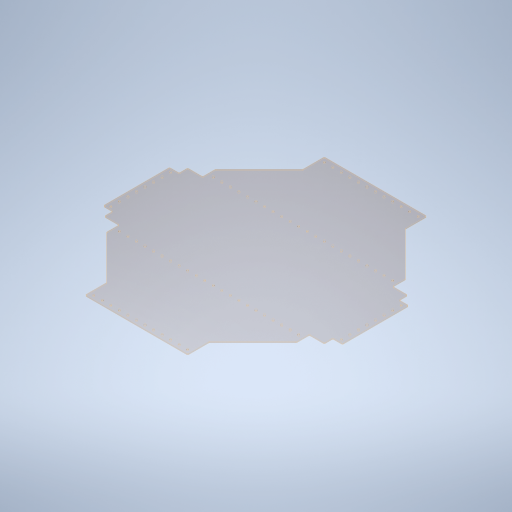
# Autodesk Inventor part: DB1-005
Saved by Autodesk Inventor 2023.4 (Build 274418000, 418)
## iProperties
Created: 2025-01-13
Part Number: DB1-005
Material: Polycarbonate, Smoke
Document SubType Name: Modeling
Designer: mavericks
Density: 1.2 g/cm^3
Appearance: Polycarbonate - Smoked
Author: mavericks
Autodesk Inventor part; units mm, degrees
ref_plane "YZ Plane" through (0, 0, 0) normal (1, 0, 0) x (0, 1, 0)
ref_plane "XZ Plane" through (0, 0, 0) normal (0, 1, 0) x (-1, 0, 0)
ref_plane "XY Plane" through (0, 0, 0) normal (0, 0, 1) x (1, 0, 0)
sketch "Sketch1" plane through (0, 0, 0) normal (0, 1, 0) x (-1, 0, 0)
  line L0 (355.6, 355.6) -> (-355.6, 355.6)
  line L1 (-355.6, 355.6) -> (-355.6, -355.6)
  line L2 (-355.6, -355.6) -> (355.6, -355.6)
  line L3 (355.6, -355.6) -> (355.6, 355.6)
  line L4 (355.6, 355.6) -> (-355.6, -355.6) construction
  line L5 (-355.6, 355.6) -> (355.6, -355.6) construction
  line L6 (152.4, 355.6) -> (152.4, 292.1)
  line L7 (152.4, 292.1) -> (292.1, 152.4)
  line L8 (292.1, 152.4) -> (355.6, 152.4)
  line L9 (-152.4, 292.1) -> (-152.4, 355.6)
  line L10 (-292.1, 152.4) -> (-152.4, 292.1)
  line L11 (-355.6, 152.4) -> (-292.1, 152.4)
  line L12 (-292.1, -152.4) -> (-355.6, -152.4)
  line L13 (-152.4, -292.1) -> (-292.1, -152.4)
  line L14 (-152.4, -355.6) -> (-152.4, -292.1)
  line L15 (152.4, -292.1) -> (152.4, -355.6)
  line L16 (292.1, -152.4) -> (152.4, -292.1)
  line L17 (355.6, -152.4) -> (292.1, -152.4)
  point P0 (0, 0)
  dimension "d0" = 711.2
  dimension "d1" = 711.2
  dimension "d2" = 63.5
  dimension "d3" = 203.2
  dimension "d6" = 360
  constraints: 36 end point, 4 perpendicular, 2 midpoint, 2 parallel, 2 point on line, 1 horizontal, 1 vertical, 29 other
  measures "d0" distance of L2.end L1.end
  measures "d1" distance of L1.end L0.end
  measures "d2" distance of L6.end L6.start
  measures "d3" distance of L0.start L6.start
extrude "Extrusion1" add sketch "Sketch1" along normal blind 3.175 contours L6 L7 L8 L3 L17 L16 L15 L2 L14 L13 L12 L1 L11 L10 L9 L0
sketch "Sketch2" plane through (0, 3.175, 0) normal (0, 1, 0) x (1, 0, 0)
  line L0 (-355.6, 152.4) -> (-355.6, -152.4) construction
  line L1 (152.4, 355.6) -> (-152.4, 355.6) construction
  line L2 (-152.4, -355.6) -> (152.4, -355.6) construction
  line L3 (355.6, -152.4) -> (355.6, 152.4) construction
  line L4 (-292.1, 152.4) -> (-355.6, 152.4) construction
  line L5 (-152.4, -292.1) -> (-152.4, -355.6) construction
  point P0 (0, 0)
  point P1 (-139.7, -342.9)
  point P2 (-139.7, 342.9)
  point P3 (342.9, 139.7)
  point P4 (-342.9, 139.7)
  point P5 (-114.3, -342.9)
  point P6 (-114.3, 342.9)
  point P7 (-88.9, -342.9)
  point P8 (-88.9, 342.9)
  point P9 (-63.5, -342.9)
  point P10 (-63.5, 342.9)
  point P11 (-38.1, -342.9)
  point P12 (-38.1, 342.9)
  point P13 (-12.7, -342.9)
  point P14 (-12.7, 342.9)
  point P15 (12.7, -342.9)
  point P16 (12.7, 342.9)
  point P17 (38.1, -342.9)
  point P18 (38.1, 342.9)
  point P19 (63.5, -342.9)
  point P20 (63.5, 342.9)
  point P21 (88.9, -342.9)
  point P22 (88.9, 342.9)
  point P23 (114.3, -342.9)
  point P24 (114.3, 342.9)
  point P25 (139.7, -342.9)
  point P26 (139.7, 342.9)
  point P27 (-342.9, 114.3)
  point P28 (342.9, 114.3)
  point P29 (-342.9, 88.9)
  point P30 (342.9, 88.9)
  point P31 (-342.9, 63.5)
  point P32 (342.9, 63.5)
  point P33 (-342.9, 38.1)
  point P34 (342.9, 38.1)
  point P35 (-342.9, 12.7)
  point P36 (342.9, 12.7)
  point P37 (-342.9, -12.7)
  point P38 (342.9, -12.7)
  point P39 (-342.9, -38.1)
  point P40 (342.9, -38.1)
  point P41 (-342.9, -63.5)
  point P42 (342.9, -63.5)
  point P43 (-342.9, -88.9)
  point P44 (342.9, -88.9)
  point P45 (-342.9, -114.3)
  point P46 (342.9, -114.3)
  point P47 (-342.9, -139.7)
  point P48 (342.9, -139.7)
  dimension "d10" = 12.7
  dimension "d11" = 12.7
  dimension "d12" = 12.7
  dimension "d13" = 12.7
  dimension "d14" = 12.7
  dimension "d15" = 12.7
  dimension "d18" = 25.4
  dimension "d25" = 25.4
  constraints: 1 horizontal, 1 horizontal alignment, 1 vertical, 1 vertical alignment, 44 other
  measures "d10" distance from line of L0 point (-342.9, 139.7)
  measures "d11" distance from line of L1 point (-139.7, 342.9)
  measures "d12" distance from line of L2 point (-139.7, -342.9)
  measures "d13" distance from line of L3 point (342.9, 139.7)
  measures "d14" distance from line of L4 point (-342.9, 139.7)
  measures "d15" distance from line of L5 point (-139.7, -342.9)
  measures "d18" distance of point (-139.7, -342.9) point (-114.3, -342.9)
  measures "d25" distance of point (-342.9, 139.7) point (-342.9, 114.3)
hole "Hole1" at (-139.7, 3.175, 342.9) at (-139.7, 3.175, -342.9) at (342.9, 3.175, -139.7) at (-342.9, 3.175, -139.7) at (-114.3, 3.175, 342.9) at (-114.3, 3.175, -342.9) at (-88.9, 3.175, 342.9) at (-88.9, 3.175, -342.9) at (-63.5, 3.175, 342.9) at (-63.5, 3.175, -342.9) at (-38.1, 3.175, 342.9) at (-38.1, 3.175, -342.9) at (-12.7, 3.175, 342.9) at (-12.7, 3.175, -342.9) at (12.7, 3.175, 342.9) at (12.7, 3.175, -342.9) at (38.1, 3.175, 342.9) at (38.1, 3.175, -342.9) at (63.5, 3.175, 342.9) at (63.5, 3.175, -342.9) at (88.9, 3.175, 342.9) at (88.9, 3.175, -342.9) at (114.3, 3.175, 342.9) at (114.3, 3.175, -342.9) at (139.7, 3.175, 342.9) at (139.7, 3.175, -342.9) at (-342.9, 3.175, -114.3) at (342.9, 3.175, -114.3) at (-342.9, 3.175, -88.9) at (342.9, 3.175, -88.9) at (-342.9, 3.175, -63.5) at (342.9, 3.175, -63.5) at (-342.9, 3.175, -38.1) at (342.9, 3.175, -38.1) at (-342.9, 3.175, -12.7) at (342.9, 3.175, -12.7) at (-342.9, 3.175, 12.7) at (342.9, 3.175, 12.7) at (-342.9, 3.175, 38.1) at (342.9, 3.175, 38.1) at (-342.9, 3.175, 63.5) at (342.9, 3.175, 63.5) at (-342.9, 3.175, 88.9) at (342.9, 3.175, 88.9) at (-342.9, 3.175, 114.3) at (342.9, 3.175, 114.3) at (-342.9, 3.175, 139.7) at (342.9, 3.175, 139.7) direction (0, -1, 0) diameter 5.1054 end through all clearance for "Flat Head Machine Screw (82)" size "#10" standard "Ansi Unified Screw Threads"
sketch "Sketch3" plane through (0, 3.175, 0) normal (0, 1, 0) x (1, 0, 0)
  circle A0 centre (-342.9, -139.7) radius 2.5527 construction
  circle A1 centre (-342.9, -114.3) radius 2.5527 construction
  circle A2 centre (-342.9, -88.9) radius 2.5527 construction
  circle A3 centre (-342.9, -63.5) radius 2.5527 construction
  circle A4 centre (-342.9, -38.1) radius 2.5527 construction
  circle A5 centre (-342.9, -12.7) radius 2.5527 construction
  circle A6 centre (-342.9, 12.7) radius 2.5527 construction
  circle A7 centre (-342.9, 38.1) radius 2.5527 construction
  circle A8 centre (-342.9, 63.5) radius 2.5527 construction
  circle A9 centre (-342.9, 88.9) radius 2.5527 construction
  circle A10 centre (-342.9, 114.3) radius 2.5527 construction
  circle A11 centre (139.7, -342.9) radius 2.5527 construction
  circle A12 centre (114.3, -342.9) radius 2.5527 construction
  circle A13 centre (88.9, -342.9) radius 2.5527 construction
  circle A14 centre (63.5, -342.9) radius 2.5527 construction
  circle A15 centre (38.1, -342.9) radius 2.5527 construction
  circle A16 centre (12.7, -342.9) radius 2.5527 construction
  circle A17 centre (-12.7, -342.9) radius 2.5527 construction
  circle A18 centre (-38.1, -342.9) radius 2.5527 construction
  circle A19 centre (-63.5, -342.9) radius 2.5527 construction
  circle A20 centre (-88.9, -342.9) radius 2.5527 construction
  circle A21 centre (-114.3, -342.9) radius 2.5527 construction
  circle A22 centre (342.9, 139.7) radius 2.5527 construction
  circle A23 centre (-139.7, -342.9) radius 2.5527 construction
  circle A24 centre (-139.7, 342.9) radius 2.5527 construction
  circle A25 centre (-342.9, 139.7) radius 2.5527 construction
  circle A26 centre (-114.3, 342.9) radius 2.5527 construction
  circle A27 centre (-88.9, 342.9) radius 2.5527 construction
  circle A28 centre (-63.5, 342.9) radius 2.5527 construction
  circle A29 centre (-38.1, 342.9) radius 2.5527 construction
  circle A30 centre (-12.7, 342.9) radius 2.5527 construction
  circle A31 centre (12.7, 342.9) radius 2.5527 construction
  circle A32 centre (38.1, 342.9) radius 2.5527 construction
  circle A33 centre (63.5, 342.9) radius 2.5527 construction
  circle A34 centre (88.9, 342.9) radius 2.5527 construction
  circle A35 centre (114.3, 342.9) radius 2.5527 construction
  circle A36 centre (139.7, 342.9) radius 2.5527 construction
  circle A37 centre (342.9, 114.3) radius 2.5527 construction
  circle A38 centre (342.9, 88.9) radius 2.5527 construction
  circle A39 centre (342.9, 63.5) radius 2.5527 construction
  circle A40 centre (342.9, 38.1) radius 2.5527 construction
  circle A41 centre (342.9, 12.7) radius 2.5527 construction
  circle A42 centre (342.9, -12.7) radius 2.5527 construction
  circle A43 centre (342.9, -38.1) radius 2.5527 construction
  circle A44 centre (342.9, -63.5) radius 2.5527 construction
  circle A45 centre (342.9, -88.9) radius 2.5527 construction
  circle A46 centre (342.9, -114.3) radius 2.5527 construction
  circle A47 centre (342.9, -139.7) radius 2.5527 construction
  line L0 (-152.4, -292.1) -> (-152.4, -355.6) construction
  line L1 (-152.4, -355.6) -> (152.4, -355.6) construction
  line L2 (152.4, -355.6) -> (152.4, -292.1) construction
  line L3 (152.4, -292.1) -> (292.1, -152.4) construction
  line L4 (292.1, -152.4) -> (355.6, -152.4) construction
  line L5 (355.6, -152.4) -> (355.6, 152.4) construction
  line L6 (355.6, 152.4) -> (292.1, 152.4) construction
  line L7 (292.1, 152.4) -> (152.4, 292.1) construction
  line L8 (152.4, 292.1) -> (152.4, 355.6) construction
  line L9 (152.4, 355.6) -> (-152.4, 355.6) construction
  line L10 (-152.4, 355.6) -> (-152.4, 292.1) construction
  line L11 (-152.4, 292.1) -> (-292.1, 152.4) construction
  line L12 (-292.1, 152.4) -> (-355.6, 152.4) construction
  line L13 (-355.6, 152.4) -> (-355.6, -152.4) construction
  line L14 (-355.6, -152.4) -> (-292.1, -152.4) construction
  line L15 (-292.1, -152.4) -> (-152.4, -292.1) construction
  line L16 (-355.6, 152.4) -> (-355.6, -152.4) construction
  line L17 (-355.6, -152.4) -> (-355.6, -98.425)
  line L18 (-355.6, -98.425) -> (-327.025, -98.425)
  line L19 (-327.025, -98.425) -> (-327.025, -123.825)
  line L20 (-327.025, -123.825) -> (-282.575, -123.825)
  line L21 (-355.6, -152.4) -> (-292.1, -152.4) construction
  line L22 (-355.6, -152.4) -> (-282.575, -152.4)
  line L23 (-282.575, -152.4) -> (-282.575, -123.825)
  line L24 (0, 0) -> (-355.6, 0) construction
  line L25 (0, 0) -> (0, 355.6) construction
  line L26 (152.4, 355.6) -> (-152.4, 355.6) construction
  circle A48 centre (-342.9, 139.7) radius 2.5527 construction
  circle A49 centre (-342.9, 114.3) radius 2.5527 construction
  circle A50 centre (-342.9, 88.9) radius 2.5527 construction
  line L27 (-355.6, 152.4) -> (-292.1, 152.4) construction
  line L28 (-355.6, 152.4) -> (-355.6, 98.425)
  line L29 (-355.6, 98.425) -> (-327.025, 98.425)
  line L30 (-327.025, 98.425) -> (-327.025, 123.825)
  line L31 (-327.025, 123.825) -> (-282.575, 123.825)
  line L32 (-355.6, 152.4) -> (-292.1, 152.4) construction
  line L33 (-355.6, 152.4) -> (-282.575, 152.4)
  line L34 (-282.575, 152.4) -> (-282.575, 123.825)
  circle A51 centre (342.9, -139.7) radius 2.5527 construction
  circle A52 centre (342.9, -114.3) radius 2.5527 construction
  circle A53 centre (342.9, -88.9) radius 2.5527 construction
  circle A54 centre (342.9, -63.5) radius 2.5527 construction
  circle A55 centre (342.9, -38.1) radius 2.5527 construction
  circle A56 centre (342.9, -12.7) radius 2.5527 construction
  circle A57 centre (342.9, 12.7) radius 2.5527 construction
  circle A58 centre (342.9, 38.1) radius 2.5527 construction
  circle A59 centre (342.9, 63.5) radius 2.5527 construction
  circle A60 centre (342.9, 88.9) radius 2.5527 construction
  circle A61 centre (342.9, 114.3) radius 2.5527 construction
  circle A62 centre (342.9, 139.7) radius 2.5527 construction
  line L35 (292.1, 152.4) -> (355.6, 152.4) construction
  line L36 (355.6, 152.4) -> (355.6, -152.4) construction
  line L37 (355.6, -152.4) -> (292.1, -152.4) construction
  line L38 (355.6, 152.4) -> (355.6, -152.4) construction
  line L39 (355.6, -152.4) -> (355.6, -98.425)
  line L40 (355.6, -98.425) -> (327.025, -98.425)
  line L41 (327.025, -98.425) -> (327.025, -123.825)
  line L42 (327.025, -123.825) -> (282.575, -123.825)
  line L43 (355.6, -152.4) -> (292.1, -152.4) construction
  line L44 (355.6, -152.4) -> (282.575, -152.4)
  line L45 (282.575, -152.4) -> (282.575, -123.825)
  circle A63 centre (342.9, 139.7) radius 2.5527 construction
  circle A64 centre (342.9, 114.3) radius 2.5527 construction
  line L46 (355.6, 152.4) -> (355.6, 98.425)
  circle A65 centre (342.9, 88.9) radius 2.5527 construction
  line L47 (355.6, 98.425) -> (327.025, 98.425)
  line L48 (327.025, 98.425) -> (327.025, 123.825)
  line L49 (355.6, 152.4) -> (282.575, 152.4)
  line L50 (327.025, 123.825) -> (282.575, 123.825)
  line L51 (282.575, 152.4) -> (282.575, 123.825)
  line L52 (355.6, 152.4) -> (292.1, 152.4) construction
  line L53 (355.6, 152.4) -> (292.1, 152.4) construction
  line L54 (-282.575, -152.4) -> (-282.575, -161.925)
  line L55 (-292.1, -152.4) -> (-152.4, -292.1) construction
  line L56 (-282.575, -161.925) -> (-292.1, -152.4)
  line L57 (-282.575, 152.4) -> (-282.575, 161.925)
  line L58 (-282.575, 161.925) -> (-292.1, 152.4)
  line L59 (282.575, -152.4) -> (282.575, -161.925)
  line L60 (282.575, -161.925) -> (292.1, -152.4)
  line L61 (282.575, 152.4) -> (282.575, 161.925)
  line L62 (282.575, 161.925) -> (292.1, 152.4)
  point P0 (355.6, 0)
  dimension "d39" = 53.975
  dimension "d40" = 28.575
  dimension "d42" = 28.575
  dimension "d43" = 73.025
  constraints: 86 end point, 37 symmetric about line, 18 centre point, 3 point on line, 2 collinear, 2 horizontal, 2 midpoint, 2 perpendicular, 1 vertical, 18 other
  measures "d39" distance of L13.end L17.end
  measures "d40" distance of L17.end L18.end
  measures "d42" distance between parallel lines of L14 L20
  measures "d43" distance from line of L17 L20.end
extrude "Extrusion2" cut sketch "Sketch3" against normal through all
fillet "Fillet1" radius 3.302 28 edges at (-152.4, 1.5875, 355.6) (-152.4, 1.5875, 292.1) (-282.575, 1.5875, 161.925) (-282.575, 1.5875, 123.825) (-327.025, 1.5875, 98.425) (-327.025, 1.5875, 123.825) (-355.6, 1.5875, 98.425) (-355.6, 1.5875, -98.425) (-327.025, 1.5875, -98.425) (-327.025, 1.5875, -123.825) (-282.575, 1.5875, -123.825) (-282.575, 1.5875, -161.925) (-152.4, 1.5875, -292.1) (-152.4, 1.5875, -355.6) (152.4, 1.5875, -292.1) (152.4, 1.5875, -355.6) (282.575, 1.5875, -161.925) (282.575, 1.5875, -123.825) (327.025, 1.5875, -123.825) (327.025, 1.5875, -98.425) (355.6, 1.5875, -98.425) (355.6, 1.5875, 98.425) (327.025, 1.5875, 98.425) (327.025, 1.5875, 123.825) (282.575, 1.5875, 123.825) (282.575, 1.5875, 161.925) (152.4, 1.5875, 292.1) (152.4, 1.5875, 355.6)
sketch "Sketch4" plane through (0, 3.175, 0) normal (0, 1, 0) x (1, 0, 0)
  line L0 (149.098, 355.6) -> (-149.098, 355.6) construction
  line L1 (-149.098, -355.6) -> (149.098, -355.6) construction
  line L2 (355.6, -95.123) -> (355.6, 95.123) construction
  point P0 (0, 0)
  point P1 (266.7, 139.7)
  point P2 (266.7, -139.7)
  point P3 (241.3, 139.7)
  point P4 (241.3, -139.7)
  point P5 (215.9, 139.7)
  point P6 (215.9, -139.7)
  point P7 (190.5, 139.7)
  point P8 (190.5, -139.7)
  point P9 (165.1, 139.7)
  point P10 (165.1, -139.7)
  point P11 (139.7, 139.7)
  point P12 (139.7, -139.7)
  point P13 (114.3, 139.7)
  point P14 (114.3, -139.7)
  point P15 (88.9, 139.7)
  point P16 (88.9, -139.7)
  point P17 (63.5, 139.7)
  point P18 (63.5, -139.7)
  point P19 (38.1, 139.7)
  point P20 (38.1, -139.7)
  point P21 (12.7, 139.7)
  point P22 (12.7, -139.7)
  point P23 (-12.7, 139.7)
  point P24 (-12.7, -139.7)
  point P25 (-38.1, 139.7)
  point P26 (-38.1, -139.7)
  point P27 (-63.5, 139.7)
  point P28 (-63.5, -139.7)
  point P29 (-88.9, 139.7)
  point P30 (-88.9, -139.7)
  point P31 (-114.3, 139.7)
  point P32 (-114.3, -139.7)
  point P33 (-139.7, 139.7)
  point P34 (-139.7, -139.7)
  point P35 (-165.1, 139.7)
  point P36 (-165.1, -139.7)
  point P37 (-190.5, 139.7)
  point P38 (-190.5, -139.7)
  point P39 (-215.9, 139.7)
  point P40 (-215.9, -139.7)
  point P41 (-241.3, 139.7)
  point P42 (-241.3, -139.7)
  point P43 (-266.7, 139.7)
  point P44 (-266.7, -139.7)
  dimension "d45" = 215.9
  dimension "d46" = 215.9
  dimension "d47" = 88.9
  dimension "d50" = 25.4
  constraints: 1 horizontal, 1 vertical alignment, 42 other
  measures "d45" distance from line of L0 point (266.7, 139.7)
  measures "d46" distance from line of L1 point (266.7, -139.7)
  measures "d47" distance from line of point (266.7, 139.7) L2
  measures "d50" distance of point (266.7, 139.7) point (241.3, 139.7)
hole "Hole2" at (266.7, 3.175, -139.7) at (266.7, 3.175, 139.7) at (241.3, 3.175, -139.7) at (241.3, 3.175, 139.7) at (215.9, 3.175, -139.7) at (215.9, 3.175, 139.7) at (190.5, 3.175, -139.7) at (190.5, 3.175, 139.7) at (165.1, 3.175, -139.7) at (165.1, 3.175, 139.7) at (139.7, 3.175, -139.7) at (139.7, 3.175, 139.7) at (114.3, 3.175, -139.7) at (114.3, 3.175, 139.7) at (88.9, 3.175, -139.7) at (88.9, 3.175, 139.7) at (63.5, 3.175, -139.7) at (63.5, 3.175, 139.7) at (38.1, 3.175, -139.7) at (38.1, 3.175, 139.7) at (12.7, 3.175, -139.7) at (12.7, 3.175, 139.7) at (-12.7, 3.175, -139.7) at (-12.7, 3.175, 139.7) at (-38.1, 3.175, -139.7) at (-38.1, 3.175, 139.7) at (-63.5, 3.175, -139.7) at (-63.5, 3.175, 139.7) at (-88.9, 3.175, -139.7) at (-88.9, 3.175, 139.7) at (-114.3, 3.175, -139.7) at (-114.3, 3.175, 139.7) at (-139.7, 3.175, -139.7) at (-139.7, 3.175, 139.7) at (-165.1, 3.175, -139.7) at (-165.1, 3.175, 139.7) at (-190.5, 3.175, -139.7) at (-190.5, 3.175, 139.7) at (-215.9, 3.175, -139.7) at (-215.9, 3.175, 139.7) at (-241.3, 3.175, -139.7) at (-241.3, 3.175, 139.7) at (-266.7, 3.175, -139.7) at (-266.7, 3.175, 139.7) direction (0, -1, 0) diameter 5.1054 end through all clearance for "Flat Head Machine Screw (82)" size "#10" standard "Ansi Unified Screw Threads"
body "Solid1"
